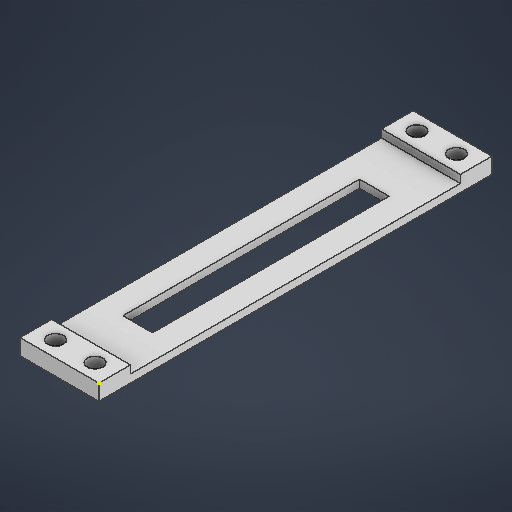
# Autodesk Inventor part: servo2servo_support
Saved by Autodesk Inventor 2026.1 (Build 301233000, 233)
## iProperties
Created: 2026-03-10
Part Number: servo2servo_support
Material: Generic
Document SubType Name: Modeling
Designer: emanuel
Density: 1 g/cm^3
Appearance: Default
Author: emanuel
Autodesk Inventor part; units mm, degrees
ref_plane "YZ Plane" through (0, 0, 0) normal (1, 0, 0) x (0, 1, 0)
ref_plane "XZ Plane" through (0, 0, 0) normal (0, 1, 0) x (-1, 0, 0)
ref_plane "XY Plane" through (0, 0, 0) normal (0, 0, 1) x (1, 0, 0)
sketch "Sketch1" plane through (0, 0, 0) normal (0, 1, 0) x (-1, 0, 0)
  line L0 (0, 0) -> (20, 0)
  line L1 (20, 0) -> (20, -99.7)
  line L2 (20, -99.7) -> (0, -99.7)
  line L3 (0, -99.7) -> (0, 0)
  line L4 (0, 0) -> (5, 0)
  line L5 (5, 0) -> (5, -4)
  line L6 (5, -4) -> (0, -4)
  line L7 (0, -4) -> (0, 0)
  line L8 (0, -99.7) -> (5, -99.7)
  line L9 (5, -99.7) -> (5, -95.7)
  line L10 (5, -95.7) -> (0, -95.7)
  line L11 (0, -95.7) -> (0, -99.7)
  line L12 (5, -4) -> (15, -4)
  line L13 (5, -95.7) -> (15, -95.7)
  circle A0 centre (15, -4) radius 2
  circle A1 centre (5, -4) radius 2
  circle A2 centre (15, -95.7) radius 2
  circle A3 centre (5, -95.7) radius 2
  dimension "d0" = 20
  dimension "d1" = 99.7
  dimension "d2" = 5
  dimension "d3" = 4
  dimension "d4" = 5
  dimension "d5" = 4
  dimension "d6" = 10
  dimension "d7" = 10
  dimension "d8" = 4
  dimension "d9" = 4
  dimension "d10" = 4
  dimension "d11" = 4
  constraints: 28 end point, 6 parallel, 5 horizontal, 4 centre point, 3 perpendicular, 1 coincident
  measures "d0" distance of L1.end L2.end
  measures "d1" distance of L0.end L1.end
  measures "d2" distance of L5.end L6.end
  measures "d3" distance of L4.end L5.end
  measures "d4" distance of L10.end L9.end
  measures "d5" distance of L9.end L8.end
  measures "d6" distance of L5.end L12.end
  measures "d7" distance of L9.end L13.end
  measures "d8" diameter of A0
  measures "d9" diameter of A1
  measures "d10" diameter of A2
  measures "d11" diameter of A3
extrude "Extrusion1" add sketch "Sketch1" along normal blind 4 contours L0 L5 A1 L6 L3 | L0 L1 L2 L9 A3 L10 L3 L6 A1 L5 | L10 A3 L9 L2 L3
sketch "Sketch2" plane through (0, 4, 0) normal (0, 1, 0) x (1, 0, 0)
  line L0 (-20, 99.7) -> (-20, 0) projected
  line L1 (0, 0) -> (0, 99.7) projected
  line L2 (-20, 0) -> (0, 0)
  line L3 (0, 0) -> (0, 8)
  line L4 (0, 8) -> (-20, 8)
  line L5 (-20, 8) -> (-20, 0)
  line L6 (0, 99.7) -> (-20, 99.7) projected
  line L7 (-20, 99.7) -> (0, 99.7)
  line L8 (0, 99.7) -> (0, 91.7)
  line L9 (0, 91.7) -> (-20, 91.7)
  line L10 (-20, 91.7) -> (-20, 99.7)
  line L11 (-20, 91.7) -> (0, 91.7)
  line L12 (0, 91.7) -> (0, 8)
  line L13 (0, 8) -> (-20, 8)
  line L14 (-20, 8) -> (-20, 91.7)
  dimension "d14" = 8
  dimension "d15" = 8
  constraints: 24 end point, 6 parallel, 3 horizontal, 3 perpendicular, 2 point on line
  measures "d14" distance of L3.end L2.end
  measures "d15" distance of L7.end L8.end
sketch "Sketch3" plane through (0, 4, 0) normal (0, 1, 0) x (1, 0, 0)
  point P0 (0, 0)
extrude "Extrusion2" cut sketch "Sketch2" against normal blind 2 contours L9 L1 L4 L0
sketch "Sketch4" plane through (0, 2, 0) normal (0, 1, 0) x (1, 0, 0)
  line L0 (-20, 8) -> (-20, 91.7) projected
  line L1 (-20, 49.85) -> (-10, 49.85)
  line L2 (-13.75, 19.85) -> (-6.25, 19.85)
  line L3 (-6.25, 19.85) -> (-6.25, 79.85)
  line L4 (-6.25, 79.85) -> (-13.75, 79.85)
  line L5 (-13.75, 79.85) -> (-13.75, 19.85)
  line L6 (-13.75, 19.85) -> (-6.25, 79.85) construction
  line L7 (-6.25, 19.85) -> (-13.75, 79.85) construction
  point P0 (0, 0)
  dimension "d18" = 10
  dimension "d19" = 7.5
  dimension "d20" = 60
  constraints: 14 end point, 3 midpoint, 2 horizontal, 2 parallel, 1 perpendicular
  measures "d18" distance of L1.start L1.end
  measures "d19" distance of L4.end L3.end
  measures "d20" distance of L3.end L2.end
extrude "Extrusion3" cut sketch "Sketch4" against normal blind 2
body "Solid1"
